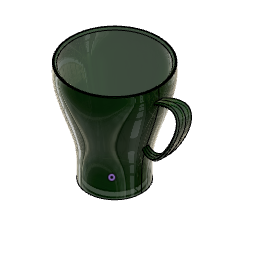
Lab01 v11 (Autodesk Fusion 360 design; units mm, degrees)
Autodesk Fusion 360 part; units mm, degrees
sketch "Sketch1" plane through (0, 0, 0) normal (0, 1, 0) x (1, 0, 0)
sketch "Sketch2" plane through (0, 0, 0) normal (0, 1, 0) x (1, 0, 0)
sketch "Sketch3" plane through (0, 0, 0) normal (0, 1, 0) x (1, 0, 0)
sketch "Sketch4" plane through (0, 0, 0) normal (0, 1, 0) x (1, 0, 0)
  line L0 (0, 0) -> (0, -3) construction
  line L1 (0, 0) -> (3, 0) construction
  line L2 (3, 0) -> (3, -3) construction
  line L3 (3, -3) -> (0, -3) construction
  line L4 (0, -3) -> (0, 0) construction
  line L5 (0, -3) -> (3, -3) construction
  line L6 (3, -3) -> (3, -6)
  line L7 (3, -6) -> (0, -6) construction
  line L8 (0, -6) -> (0, -3) construction
  line L9 (3, -3) -> (6, -3) construction
  line L10 (6, -3) -> (6, -6) construction
  line L11 (6, -6) -> (3, -6) construction
  line L12 (3, -6) -> (3, -3) construction
  line L13 (6, -3) -> (13, -3) construction
  line L14 (13, -3) -> (28, -3) construction
  line L15 (6, -6) -> (13, -6) construction
  line L16 (28, -3) -> (31, -3) construction
  line L17 (3, -6) -> (3, -16) construction
  line L18 (3, -16) -> (28, -16) construction
  line L19 (28, -16) -> (31, -16) construction
  line L20 (3, -16) -> (3, -46) construction
  line L21 (3, -46) -> (3, -91) construction
  line L22 (3, -91) -> (3, -103) construction
  line L23 (3, -91) -> (46, -91) construction
  line L24 (3, -103) -> (46, -103) construction
  line L25 (3, -46) -> (33, -46) construction
  line L26 (33, -46) -> (36, -46) construction
  line L27 (46, -91) -> (49, -91) construction
  line L28 (46, -103) -> (49, -103) construction
  line L29 (49, -103) -> (49, -106) construction
  line L30 (49, -106) -> (46, -106)
  line L31 (46, -106) -> (46, -103) construction
  line L32 (28, -3) -> (31, -3) construction
  line L33 (31, -3) -> (31, -4) construction
  line L34 (31, -4) -> (28, -4) construction
  line L35 (28, -4) -> (28, -3) construction
  line L36 (28, -3) -> (31, -3) construction
  line L37 (31, -3) -> (31, -1) construction
  line L38 (31, -1) -> (28, -1) construction
  line L39 (28, -1) -> (28, -3) construction
  line L40 (29.5, -1) -> (29.5, 0) construction
  spline S0 degree 5 poles (31, -1) (30.9992, -1.2619) (30.998, -1.7466) (30.9974, -2.3559) (30.9989, -2.9353) (31.0029, -3.3816) (31.0021, -3.9452) (30.9904, -5.0601) (30.9704, -6.8828) (30.9511, -9.3911) (30.9479, -12.4386) (30.9817, -15.8261) (31.0778, -19.3639) (31.2652, -22.9411) (31.5744, -26.5118) (32.0342, -30.0795) (32.6695, -33.6825) (33.4979, -37.3794) (34.5278, -41.2343) (35.7549, -45.302) (37.1597, -49.6143) (38.7039, -54.163) (40.3347, -58.9056) (41.9896, -63.7736) (43.6019, -68.6802) (45.1048, -73.5277) (46.4371, -78.2155) (47.5477, -82.6472) (48.4007, -86.7384) (48.9805, -90.4247) (49.2968, -93.6686) (49.3912, -96.4694) (49.3281, -98.8549) (49.1823, -100.8694) (49.0269, -102.5623) (48.9225, -103.9776) (48.9063, -104.9082) (48.9367, -105.4966) (48.9757, -105.8403) (49, -106) knots 0 0 0 0 0 0 0.028571 0.057143 0.085714 0.114286 0.142857 0.171429 0.2 0.228571 0.257143 0.285714 0.314286 0.342857 0.371429 0.4 0.428571 0.457143 0.485714 0.514286 0.542857 0.571429 0.6 0.628571 0.657143 0.685714 0.714286 0.742857 0.771429 0.8 0.828571 0.857143 0.885714 0.914286 0.942857 0.971429 1 1 1 1 1 1
  spline S1 degree 5 poles (46, -106) (45.9757, -105.8403) (45.9367, -105.4966) (45.9063, -104.9082) (45.9225, -103.9776) (46.0269, -102.5623) (46.1823, -100.8694) (46.3281, -98.8549) (46.3912, -96.4694) (46.2968, -93.6686) (45.9805, -90.4247) (45.4007, -86.7384) (44.5477, -82.6472) (43.4371, -78.2155) (42.1048, -73.5277) (40.6019, -68.6802) (38.9896, -63.7736) (37.3347, -58.9056) (35.7039, -54.163) (34.1597, -49.6143) (32.7549, -45.302) (31.5278, -41.2343) (30.4979, -37.3794) (29.6695, -33.6825) (29.0342, -30.0795) (28.5744, -26.5118) (28.2652, -22.9411) (28.0778, -19.3639) (27.9817, -15.8261) (27.9479, -12.4386) (27.9511, -9.3911) (27.9704, -6.8828) (27.9904, -5.0601) (28.0021, -3.9452) (28.0029, -3.3816) (27.9989, -2.9353) (27.9974, -2.3559) (27.998, -1.7466) (27.9992, -1.2619) (28, -1) knots 0 0 0 0 0 0 0.028571 0.057143 0.085714 0.114286 0.142857 0.171429 0.2 0.228571 0.257143 0.285714 0.314286 0.342857 0.371429 0.4 0.428571 0.457143 0.485714 0.514286 0.542857 0.571429 0.6 0.628571 0.657143 0.685714 0.714286 0.742857 0.771429 0.8 0.828571 0.857143 0.885714 0.914286 0.942857 0.971429 1 1 1 1 1 1
  spline S2 degree 5 poles (3, -6) (3.1358, -5.9942) (3.4205, -5.9843) (3.8868, -5.975) (4.5876, -5.9736) (5.5983, -5.989) (6.7474, -6.0175) (8.0366, -6.0497) (9.4656, -6.0717) (11.0332, -6.0679) (12.7369, -6.0232) (14.5726, -5.9248) (16.5337, -5.7655) (18.6129, -5.5421) (20.8025, -5.2541) (23.096, -4.9024) (25.0098, -4.5716) (26.4883, -4.2963) (27.4929, -4.1008) (28, -4) knots 0 0 0 0 0 0 0.066667 0.133333 0.2 0.266667 0.333333 0.4 0.466667 0.533333 0.6 0.666667 0.733333 0.8 0.866667 0.933333 1 1 1 1 1 1
  spline S3 degree 5 poles (3, -3) (3.1358, -2.9942) (3.4205, -2.9843) (3.8868, -2.975) (4.5876, -2.9736) (5.5983, -2.989) (6.7474, -3.0175) (8.0366, -3.0497) (9.4656, -3.0717) (11.0332, -3.0679) (12.7369, -3.0232) (14.5726, -2.9248) (16.5337, -2.7655) (18.6129, -2.5421) (20.8025, -2.2541) (23.096, -1.9024) (25.0098, -1.5716) (26.4883, -1.2963) (27.4929, -1.1008) (28, -1) knots 0 0 0 0 0 0 0.066667 0.133333 0.2 0.266667 0.333333 0.4 0.466667 0.533333 0.6 0.666667 0.733333 0.8 0.866667 0.933333 1 1 1 1 1 1
  arc A0 (31, -1) -> (28, -1) centre (29.5, -1.625) ccw
  line L41 (49, -91) -> (74, -91) construction
  line L42 (36, -46) -> (51, -46) construction
  spline S4 degree 5 poles (36, -46) (36.6394, -45.1618) (37.968, -43.7137) (40.1106, -42.2268) (43.2692, -41.6249) (47.7024, -43.1785) (52.5464, -46.9537) (57.6262, -52.6791) (62.6488, -59.857) (67.251, -67.8594) (71.0312, -75.9873) (73.5865, -83.5378) (74.5523, -89.8693) (73.6392, -94.4615) (70.694, -97.0062) (65.6752, -97.3753) (60.0137, -95.9103) (54.8581, -93.833) (51.0196, -92.0163) (49, -91) knots 0 0 0 0 0 0 0.066667 0.133333 0.2 0.266667 0.333333 0.4 0.466667 0.533333 0.6 0.666667 0.733333 0.8 0.866667 0.933333 1 1 1 1 1 1
  spline S5 degree 3 poles (33.6147, -44.1806) (35.0857, -42.2519) (36.837, -40.7453) (38.9033, -39.9029) (40.7833, -39.1365) (42.8782, -38.9842) (44.8879, -39.3968) (47.8038, -39.9955) (50.5579, -41.6531) (53.2839, -44.0042) (56.6283, -46.8886) (59.9718, -50.8966) (63.1467, -55.5281) (67.1196, -61.3238) (70.7941, -68.0664) (73.3795, -74.4054) (75.3184, -79.1596) (76.652, -83.6518) (76.9984, -87.5925) (77.2064, -89.9591) (77.0707, -92.1623) (76.3238, -94.1615) (75.7319, -95.746) (74.6968, -97.1913) (73.2979, -98.1887) (71.8169, -99.2445) (70.024, -99.7747) (68.1315, -99.9103) (65.1581, -100.1234) (61.8401, -99.4581) (57.9617, -98.1339) (54.8852, -97.0834) (51.4607, -95.5967) (47.6514, -93.6798) knots 0 0 0 0 0.077185 0.077185 0.077185 0.14741 0.14741 0.14741 0.249295 0.249295 0.249295 0.374298 0.374298 0.374298 0.530723 0.530723 0.530723 0.648043 0.648043 0.648043 0.718499 0.718499 0.718499 0.774343 0.774343 0.774343 0.833458 0.833458 0.833458 0.92633 0.92633 0.92633 1 1 1 1
  dimension "d14" = 3
  dimension "d15" = 3
  dimension "d16" = 3
  dimension "d17" = 3
  dimension "d18" = 3
  dimension "d19" = 3
  dimension "d20" = 3
  dimension "d21" = 7
  dimension "d22" = 15
  dimension "d23" = 7
  dimension "d24" = 3
  dimension "d44" = 10
  dimension "d45" = 25
  dimension "d46" = 3
  dimension "d47" = 30
  dimension "d48" = 45
  dimension "d49" = 12
  dimension "d50" = 43
  dimension "d51" = 43
  dimension "d52" = 30
  dimension "d53" = 3
  dimension "d54" = 3
  dimension "d55" = 3
  dimension "d56" = 3
  dimension "d57" = 3
  dimension "d58" = 1
  dimension "d59" = 3
  dimension "d60" = 2
  dimension "d61" = 1
  dimension "d63" = 25
  dimension "d64" = 15
  constraint coincident L0.start L1.start
  constraint vertical L0
  constraint horizontal L1
  constraint vertical L2
  constraint horizontal L3
  constraint vertical L4
  constraint horizontal L5
  constraint vertical L6
  constraint horizontal L7
  constraint vertical L8
  constraint horizontal L9
  constraint vertical L10
  constraint horizontal L11
  constraint vertical L12
  constraint perpendicular L10 L13
  constraint parallel L13 L14
  constraint perpendicular L10 L15
  constraint parallel L14 L16
  constraint perpendicular L7 L17
  constraint perpendicular L17 L18
  constraint parallel L18 L19
  constraint perpendicular L18 L20
  constraint parallel L20 L21
  constraint parallel L21 L22
  constraint perpendicular L22 L23
  constraint perpendicular L22 L24
  constraint perpendicular L20 L25
  constraint perpendicular L22 L26
  constraint horizontal L27
  constraint horizontal L28
  constraint vertical L29
  constraint horizontal L30
  constraint vertical L31
  constraint horizontal L32
  constraint vertical L33
  constraint horizontal L34
  constraint vertical L35
  constraint horizontal L36
  constraint vertical L37
  constraint horizontal L38
  constraint vertical L39
  constraint midpoint L38 L40.start
  constraint perpendicular L38 L40
  constraint coincident L34.end L35.start
  constraint coincident L40.end A0
  constraint coincident L27.end L41.start
  constraint parallel L27 L41
  constraint coincident L26.end L42.start
  constraint parallel L26 L42
  measures "d14" distance of L0.start L0.end
  measures "d15" distance of L0.start L1.end
  measures "d16" distance of L0.start L0.end
  measures "d17" distance of L0.end L2.end
  measures "d18" distance of L0.end L7.end
  measures "d19" distance of L2.end L9.end
  measures "d20" distance of L2.end L6.end
  measures "d21" distance of L9.end L13.end
  measures "d22" distance of L13.end L14.end
  measures "d23" distance of L10.end L15.end
  measures "d24" distance of L14.end L16.end
  measures "d44" distance of L6.end L17.end
  measures "d45" distance of L17.end L18.end
  measures "d46" distance of L18.end L19.end
  measures "d47" distance of L17.end L20.end
  measures "d48" distance of L20.end L21.end
  measures "d49" distance of L21.end L22.end
  measures "d50" distance of L21.end L23.end
  measures "d51" distance of L22.end L24.end
  measures "d52" distance of L20.end L25.end
  measures "d53" distance of L25.end L26.end
  measures "d54" distance of L23.end L27.end
  measures "d55" distance of L24.end L28.end
  measures "d56" distance of L24.end L30.end
  measures "d57" distance of L14.end L16.end
  measures "d58" distance of L14.end L34.end
  measures "d59" distance of L14.end L16.end
  measures "d60" distance of L14.end L38.end
  measures "d61" distance of L40.start L40.end
  measures "d63" distance of L27.end L41.end
  measures "d64" distance of L26.end L42.end
revolve "Revolve1" add sketch "Sketch4" angle 360 about axis through (3, 0, 16) along (0, 0, 1) contours L6 S1 S2 S3 | L30 S0 S1 A0 makes body 1
revolve "Revolve2" add sketch "Sketch4" angle 6 about axis through (3, 0, 46) along (0, 0, 1) second angle 6 separate body contours S0 S4 S5 makes body 2
fillet "Fillet1" radius 0.5 1 edges at (-39.8871, -16.6343, 106) on bodies 1
fillet "Fillet2" radius 1.75 1 edges at (-37.0901, -15.5495, 106) on bodies 1
fillet "Fillet3" radius 2.5 1 edges at (-20.3082, -9.0404, 4) on bodies 1
fillet "Fillet4" radius 0.75 1 faces at (23.7097, -1.163, 1.7839) on bodies 1
fillet "Fillet5" radius 1.3 4 edges at (71.6846, 7.219, 71.348) (68.6516, 6.9003, 71.8951) (71.6846, -7.219, 71.348) (68.6516, -6.9003, 71.8951) on bodies 2
equation "w = 3 mm" comment "Comment"
equation "r0 = 22 mm"
equation "r1 = 25 mm"
equation "r2 = 30 mm"
equation "r3 = 43 mm"
equation "h0 = 10 mm"
equation "h1 = 30 mm"
equation "h2 = 45 mm"
equation "h3 = 12 mm"
equation "u0 = 15 mm"
equation "u1 = 25 mm"
equation "d14 = w"
equation "d15 = w"
equation "d16 = w"
equation "d17 = w"
equation "d18 = w"
equation "d19 = w"
equation "d20 = w"
equation "d21 = n0"
equation "d22 = u0"
equation "d23 = n0"
equation "d24 = w"
equation "d44 = h0"
equation "d45 = u1"
equation "d46 = w"
equation "d47 = r2"
equation "d48 = h2"
equation "d49 = h3"
equation "d50 = r3"
equation "d51 = r3"
equation "d52 = h1"
equation "d53 = w"
equation "d54 = w"
equation "d55 = w"
equation "d56 = w"
equation "d57 = w"
equation "d58 = n1"
equation "d59 = w"
equation "d60 = n2"
equation "d61 = n1"
equation "d63 = r1"
equation "d64 = u0"
equation "d65 = -w"
equation "f0 = 0.5 mm"
equation "f1 = 1.75 mm"
equation "f2 = 2.5 mm"
equation "f3 = 0.75 mm"
equation "f4 = 1.3 mm"
equation "d74 = f0"
equation "d76 = f1"
equation "d78 = f2"
equation "d80 = f3"
equation "d82 = f4"
equation "n0 = 7 mm"
equation "n1 = 1 mm"
equation "n2 = 2 mm"
named bodies: "mug", "mug_ear"
